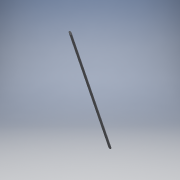
# Autodesk Inventor part: Out pipe
Saved by Autodesk Inventor 2019 (Build 230136000, 136)
## iProperties
Created: 2019-11-13
Part Number: Out pipe
Material: Generic
Document SubType Name: Modeling
Designer: Administrator
Density: 1 g/cm^3
Appearance: Default
Author: Administrator
Autodesk Inventor part; units mm, degrees
ref_plane "YZ Plane" through (0, 0, 0) normal (1, 0, 0) x (0, 1, 0)
ref_plane "XZ Plane" through (0, 0, 0) normal (0, 1, 0) x (-1, 0, 0)
ref_plane "XY Plane" through (0, 0, 0) normal (0, 0, 1) x (1, 0, 0)
sketch "Sketch1" plane through (0, 0, 0) normal (0, 0, 1) x (1, 0, 0)
  circle A0 centre (0, 0) radius 25.4
  dimension "d2" = 50.8
  constraints: 1 centre point, 1 coincident
  measures "d2" diameter of A0
sketch3d "3D Sketch1"
  line L0 (0, -11.2544, 25.1163) -> (0, 1893.7456, 660.1163)
  dimension "d6" = 1905
  dimension "d7" = 90
  dimension "d8" = 635
sweep "Sweep1" add profiles "Sketch1" path "3D Sketch1"
body "Solid1"
